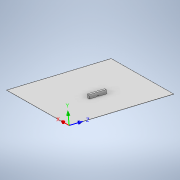
# Autodesk Inventor part: Edificio individual
Saved by Autodesk Inventor 2021 (Build 250183000, 183)
## iProperties
Created: 2021-06-11
Part Number: Edificio individual
Material: Genérico
Document SubType Name: Modeling
Designer: luise
Density: 1 g/cm^3
Appearance: Valor por defecto
Author: luise
Autodesk Inventor part; units mm, degrees
ref_plane "YZ Plane" through (0, 0, 0) normal (1, 0, 0) x (0, 1, 0)
ref_plane "XZ Plane" through (0, 0, 0) normal (0, 1, 0) x (-1, 0, 0)
ref_plane "XY Plane" through (0, 0, 0) normal (0, 0, 1) x (1, 0, 0)
sketch "Boceto8" plane through (0, 0, 0) normal (0, 1, 0) x (-1, 0, 0)
  line L0 (0, 0) -> (-480000, 0)
  line L1 (-480000, 0) -> (-480000, 480000)
  line L2 (-480000, 480000) -> (0, 480000)
  line L3 (0, 480000) -> (0, 0)
  dimension "d42" = 480000
  dimension "d43" = 480000
  constraints: 8 end point, 2 parallel, 1 horizontal, 1 perpendicular
  measures "d42" distance of L1.end L2.end
  measures "d43" distance of L0.end L1.end
sketch "Boceto9" plane through (0, 0, 0) normal (0, 1, 0) x (-1, 0, 0)
  line L0 (-180000, 280000) -> (-192000, 280000)
  line L1 (-192000, 280000) -> (-192000, 200000)
  line L2 (-192000, 200000) -> (-180000, 200000)
  line L3 (-180000, 200000) -> (-180000, 280000)
  line L4 (-480000, 0) -> (-480000, 480000) projected
  line L5 (0, 480000) -> (0, 0) projected
  line L6 (-480000, 480000) -> (0, 480000) projected
  line L7 (0, 0) -> (-480000, 0) projected
  line L8 (0, 240000) -> (-480000, 240000)
  dimension "d44" = 12000
  dimension "d45" = 80000
  dimension "d61" = 180000
  constraints: 10 end point, 2 midpoint, 2 parallel, 1 horizontal, 1 perpendicular, 1 other
  measures "d44" distance of L2.end L1.end
  measures "d45" distance of L1.end L0.end
  measures "d61" distance between parallel lines of L3 L5
extrude "Extrusión7" add sketch "Boceto9" along normal blind 18000 contours L3 L8 L1 L0 | L3 L2 L1 L8
sketch "Boceto10" plane through (192000, 0, 280000) normal (1, 0, 0) x (0, 0, -1)
  line L0 (37000, 4000) -> (43000, 4000)
  line L1 (43000, 4000) -> (43000, 0)
  line L2 (43000, 0) -> (37000, 0)
  line L3 (37000, 0) -> (37000, 4000)
  line L4 (80000, 0) -> (0, 0) projected
  line L5 (40000, 0) -> (40000, 18049)
  line L6 (0, 0) -> (80000, 0) projected
  point P0 (280000, 0)
  dimension "d49" = 6000
  dimension "d50" = 4000
  constraints: 10 end point, 2 parallel, 1 collinear, 1 horizontal, 1 midpoint, 1 perpendicular, 1 vertical, 1 other
  measures "d49" distance of L1.end L2.end
  measures "d50" distance of L0.end L1.end
extrude "Extrusión8" cut sketch "Boceto10" against normal through all
extrude "Extrusión9" add sketch "Boceto8" against normal blind 1000 separate body
